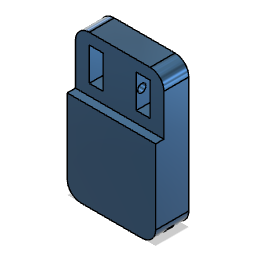
Robot Assembly Prototype v7 (Autodesk Fusion 360 archive; units mm, degrees)
design "Draft Sketch"
Autodesk Fusion 360 part; units mm, degrees
sketch "Sketch1" plane through (0, 0, 0) normal (0, 0, 1) x (1, 0, 0)
  line L0 (0, 0) -> (-320, 0)
  line L1 (-320, 0) -> (-320, 320)
  line L2 (-320, 320) -> (0, 320)
  line L3 (0, 320) -> (0, 0)
  line L4 (-320, 320) -> (-320, 470)
  line L5 (-270, 520) -> (-50, 520)
  line L6 (0, 470) -> (0, 320)
  arc A0 (-270, 520) -> (-320, 470) centre (-270, 470) ccw
  arc A1 (0, 470) -> (-50, 520) centre (-50, 470) ccw
  point P0 (-320, 520)
  dimension "d1" = 320
  dimension "d2" = 320
  dimension "d3" = 200
  dimension "d4" = 50
  dimension "d5" = 50
  constraint coincident L0.start L3.end
  constraint horizontal L0
  constraint perpendicular L0 L1
  constraint perpendicular L1 L2
  constraint perpendicular L0 L3
  constraint perpendicular L2 L4
  constraint perpendicular L4 L5
  constraint perpendicular L2 L6
  constraint coincident P0 L4
  constraint coincident P0 L5
  constraint tangent L4 A0
  constraint tangent L5 A0
  constraint tangent L5 A1
  constraint tangent L6 A1
  measures "d1" distance of L0.start L0.end
  measures "d2" distance of L0.end L1.end
  measures "d3" distance of L1.end P0
  measures "d4" radius of A0
  measures "d5" radius of A1
extrude "Extrude1" add sketch "Sketch1" along normal blind 70 contours L2 L4 L5 L6 A0 A1
extrude "Extrude2" add sketch "Sketch1" along normal blind 100 contours L0 L1 L2 L3
sketch "Sketch2" plane through (0, 0, 0) normal (1, 0, 0) x (0, 0, -1)
sketch "Sketch3" plane through (0, 0, 0) normal (1, 0, 0) x (0, 0, -1)
  line L0 (-70, 320) -> (-70, 390)
  circle A0 centre (-50, 390) radius 50
  dimension "d10" = 70
  dimension "d11" = 100
  constraint vertical L0
  measures "d10" distance of L0.start L0.end
  measures "d11" diameter of A0
extrude "Extrude3" add sketch "Sketch3" against normal blind 30
sketch "Sketch4" plane through (-320, 0, 0) normal (-1, 0, 0) x (0, 0, 1)
  line L0 (0, 470) -> (0, 0)
  line L1 (0, 0) -> (100, 0)
  line L2 (100, 0) -> (100, 320)
  line L3 (100, 320) -> (70, 320)
  line L4 (70, 320) -> (70, 470)
  line L5 (70, 470) -> (0, 470)
  line L6 (70, 320) -> (70, 390)
  circle A0 centre (50, 390) radius 50
  dimension "d14" = 70
  constraint coincident L3.end L4.start
  constraint perpendicular L3 L6
  measures "d14" distance of L3.end L6.end
extrude "Extrude4" add sketch "Sketch4" against normal blind 30 contours L4 L6 A0 picked at (89.8253, 392.4067)
delete_face "DeleteFace1" 1 faces at (-290, 381.5611, 84.673)
delete_face "DeleteFace2" 1 faces at (-10, 346.317, 74.3269)
sketch "Sketch5" plane through (0, 0, 0) normal (0, 0, 1) x (1, 0, 0)
sketch "Sketch6" plane through (0, 0, 0) normal (0, 0, 1) x (1, 0, 0)
sketch "Sketch7" plane through (0, 0, 0) normal (0, 0, 1) x (1, 0, 0)
sketch "Sketch8" plane through (0, 0, 70) normal (0, 0, 1) x (1, 0, 0)
  line L0 (-320, 320) -> (0, 320)
  line L1 (0, 320) -> (0, 470)
  arc A0 (0, 470) -> (-50, 520) centre (-50, 470) ccw
  line L2 (-50, 520) -> (-270, 520)
  arc A1 (-270, 520) -> (-320, 470) centre (-270, 470) ccw
  line L3 (-320, 470) -> (-320, 320)
  line L4 (-220, 420) -> (-220, 460)
  line L5 (-220, 460) -> (-280, 460)
  line L6 (-280, 460) -> (-280, 380)
  line L7 (-280, 380) -> (-220, 380)
  line L8 (-220, 380) -> (-220, 420)
  line L9 (-100, 420) -> (-100, 460)
  line L10 (-100, 460) -> (-40, 460)
  line L11 (-40, 460) -> (-40, 380)
  line L12 (-40, 380) -> (-100, 380)
  line L13 (-100, 380) -> (-100, 420)
  dimension "d19" = 40
  dimension "d20" = 60
  constraint perpendicular L4 L5
  constraint perpendicular L6 L7
  constraint perpendicular L9 L10
  constraint perpendicular L10 L11
  constraint perpendicular L9 L12
  measures "d19" distance of L4.start L4.end
  measures "d20" distance of L4.end L5.end
extrude "Extrude5" cut sketch "Sketch8" against normal blind 40 contours L4 L5 L6 L7 L8
extrude "Extrude6" cut sketch "Sketch8" against normal blind 40 contours L9 L10 L11 L12 L13
hole "Hole1" at (-100, 420, 50) direction (-1, 0, 0) diameter 30 depth 140 tip angle 118
extrude "Extrude7" cut 1 faces at (-80, 433.3333, 30) along direction (0, 0, -1) blind 10
extrude "Extrude8" cut 1 faces at (-240, 406.6667, 30) along direction (0, 0, -1) blind 10
sketch "Sketch9" plane through (0, 520, 0) normal (0, 1, 0) x (-1, 0, 0)
  line L0 (50, 0) -> (270, 0)
  line L1 (270, 0) -> (270, 70)
  line L2 (270, 70) -> (50, 70)
  line L3 (50, 70) -> (50, 0)
  line L4 (172, 35) -> (172, 23)
  line L5 (172, 35) -> (172, 47)
  line L6 (172, 47) -> (148, 47)
  line L7 (148, 47) -> (148, 23)
  line L8 (148, 23) -> (172, 23)
sketch "Sketch10" plane through (0, 0, 0) normal (0, 0, 1) x (1, 0, 0)
sketch "Sketch11" plane through (0, 520, 0) normal (0, 1, 0) x (-1, 0, 0)
  line L0 (50, 0) -> (270, 0)
  line L1 (270, 0) -> (270, 70)
  line L2 (270, 70) -> (50, 70)
  line L3 (50, 70) -> (50, 0)
sketch "Sketch12" plane through (0, 520, 0) normal (0, 1, 0) x (-1, 0, 0)
fillet "Fillet1" radius 50 1 edges at (0, 0, 50)
fillet "Fillet2" radius 50 1 edges at (-320, 0, 50)
extrude "Extrude10" add sketch "Sketch1" against normal blind 20 contours L2 L4 L5 L6 A0 A1
extrude "Extrude11" add 1 faces at (-223.3333, 203.5956, 0) along direction (0, 0, -1) blind 20
extrude "Extrude12" cut 1 faces at (-240, 406.6667, 20) along direction (0, 0, -1) blind 30
extrude "Extrude13" cut 1 faces at (-80, 433.3333, 20) along direction (0, 0, -1) blind 30
extrude "Extrude14" cut 1 faces at (-240, 460, 43.3333) along direction (0, 1, 0) blind 20
extrude "Extrude15" cut 1 faces at (-260, 380, 43.3333) along direction (0, -1, 0) blind 20
extrude "Extrude16" cut 1 faces at (-80, 460, 43.3333) along direction (0, 1, 0) blind 20
extrude "Extrude17" cut 1 faces at (-60, 380, 43.3333) along direction (0, -1, 0) blind 20
sketch "Sketch13" plane through (0, 0, 0) normal (0, 1, 0) x (1, 0, 0)
  line L0 (-160, -52) -> (-148, -52)
  line L1 (-148, -52) -> (-148, -28)
  line L2 (-148, -28) -> (-172, -28)
  line L3 (-172, -28) -> (-172, -52)
  line L4 (-172, -52) -> (-160, -52)
  dimension "d91" = 12
  dimension "d92" = 24
  dimension "d93" = 24
  dimension "d94" = 24
  dimension "d95" = 12
  constraint perpendicular L0 L1
  constraint perpendicular L1 L2
  constraint perpendicular L0 L3
  constraint perpendicular L1 L4
  measures "d91" distance of L0.start L0.end
  measures "d92" distance of L0.end L1.end
  measures "d93" distance of L1.end L2.end
  measures "d94" distance of L2.end L3.end
  measures "d95" distance of L3.end L0.start
extrude "Extrude18" cut sketch "Sketch13" along normal blind 10
ref_plane "WorkPlane1" through (-9.8857, 20.153, 31.144) normal (0.802286, -0.59694, 0) x (-0.59694, -0.802286, 0)
sketch "Sketch14" plane through (-9.8857, 20.153, 31.144) normal (0.802286, -0.59694, 0) x (-0.59694, -0.802286, 0)
  line L0 (5, -20) -> (-7, -20)
  line L1 (-7, -20) -> (-7, 4)
  line L2 (-7, 4) -> (17, 4)
  line L3 (17, 4) -> (17, -20)
  line L4 (17, -20) -> (5, -20)
  dimension "d102" = 12
  dimension "d103" = 24
  dimension "d104" = 24
  dimension "d105" = 24
  dimension "d106" = 12
  constraint perpendicular L1 L2
  measures "d102" distance of L0.start L0.end
  measures "d103" distance of L0.end L1.end
  measures "d104" distance of L1.end L2.end
  measures "d105" distance of L2.end L3.end
  measures "d106" distance of L3.end L0.start
extrude "Extrude19" cut sketch "Sketch14" against normal blind 10
ref_plane "WorkPlane2" through (-307.0527, 16.4278, 56.3835) normal (-0.741055, -0.671444, 0) x (-0.671444, 0.741055, 0)
sketch "Sketch15" plane through (-307.0527, 16.4278, 56.3835) normal (-0.741055, -0.671444, 0) x (-0.671444, 0.741055, 0)
  line L0 (10.5209, 16.4074) -> (10.5209, 4.4074)
  line L1 (10.5209, 4.4074) -> (-13.4791, 4.4074)
  line L2 (-13.4791, 4.4074) -> (-13.4791, 28.4074)
  line L3 (-13.4791, 28.4074) -> (10.5209, 28.4074)
  line L4 (10.5209, 28.4074) -> (10.5209, 16.4074)
  dimension "d113" = 12
  dimension "d114" = 24
  dimension "d115" = 24
  dimension "d116" = 24
  dimension "d117" = 12
  measures "d113" distance of L0.start L0.end
  measures "d114" distance of L0.end L1.end
  measures "d115" distance of L1.end L2.end
  measures "d116" distance of L2.end L3.end
  measures "d117" distance of L3.end L0.start
extrude "Extrude20" cut sketch "Sketch15" against normal blind 10
extrude "Extrude21" add 1 faces at (-280, 440, 43.3333) along direction (1, 0, 0) blind 10
extrude "Extrude22" add 1 faces at (-40, 440, 43.3333) along direction (-1, 0, 0) blind 10
move_body "Move1" bodies 1 to x (1, 0, 0) y (0, 1, 0) z (0, 0, 1) at (160, 0, -100)
move_body "Move2" bodies 1 to x (1, 0, 0) y (0, 1, 0) z (0, 0, 1) at (0, 0, 60)

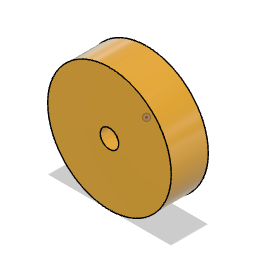
design "Wheel"
Autodesk Fusion 360 part; units mm, degrees
sketch "Sketch1" plane through (0, 0, 0) normal (0, 0, 1) x (1, 0, 0)
  circle A0 centre (0, 0) radius 7.5
  dimension "d2" = 15
  measures "d2" diameter of A0
sketch "Sketch2" plane through (0, 0, 0) normal (0, 0, 1) x (1, 0, 0)
sketch "Sketch3" plane through (0, 0, 0) normal (0, 0, 1) x (1, 0, 0)
  circle A0 centre (0, 0) radius 30
  dimension "d4" = 60
  constraint coincident A0.centre origin
  measures "d4" diameter of A0
extrude "Extrude1" add sketch "Sketch3" along normal blind 5
extrude "Extrude2" cut sketch "Sketch1" along normal blind 5
sketch "Sketch4" plane through (0, 0, 5) normal (0, 0, 1) x (1, 0, 0)
  circle A0 centre (0, 0) radius 7.5
  circle A1 centre (0, 0) radius 30
extrude "Extrude3" add sketch "Sketch4" along normal blind 5
extrude "Extrude4" add 1 faces at (22.3604, -1.863, 10) along direction (0, 0, 1) blind 5
sketch "Sketch5" plane through (0, 0, 15) normal (0, 0, 1) x (1, 0, 0)
  circle A0 centre (0, 0) radius 7.5
  circle A1 centre (0, 0) radius 30
  circle A2 centre (0, 0) radius 50
  dimension "d13" = 100
  constraint coincident A0.centre A1.centre
  measures "d13" diameter of A2
extrude "Extrude5" add sketch "Sketch5" against normal blind 15 contours A2
extrude "Extrude6" add 1 faces at (35.6193, -2.8566, 15) along direction (0, 0, 1) blind 15

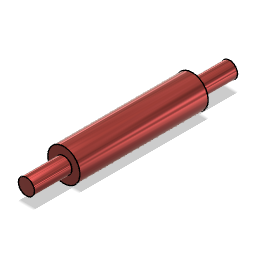
design "rod"
Autodesk Fusion 360 part; units mm, degrees
sketch "Sketch1" plane through (0, 0, 0) normal (0, 0, 1) x (1, 0, 0)
  circle A0 centre (0, 0) radius 15
  dimension "d1" = 30
  constraint coincident A0.centre origin
  measures "d1" diameter of A0
extrude "Extrude1" add sketch "Sketch1" along normal blind 120
sketch "Sketch2" plane through (0, 0, 120) normal (0, 0, 1) x (1, 0, 0)
  circle A0 centre (0, 0) radius 15
  circle A1 centre (0, 0) radius 7.5
  dimension "d4" = 15
  constraint concentric A0 A1
  measures "d4" diameter of A1
extrude "Extrude2" add sketch "Sketch2" along normal blind 10 contours A1
sketch "Sketch3" plane through (0, 0, 0) normal (0, 0, 1) x (1, 0, 0)
  circle A0 centre (0, 0) radius 7.5
  dimension "d7" = 15
  constraint coincident A0.centre origin
  measures "d7" diameter of A0
extrude "Extrude3" add sketch "Sketch3" against normal blind 10
extrude "Extrude4" add 1 faces at (1.9158, 2.8099, 130) along direction (0, 0, 1) blind 10
extrude "Extrude5" add 1 faces at (1.9158, 2.8099, -10) along direction (0, 0, -1) blind 10
extrude "Extrude6" add 1 faces at (1.9158, 2.8099, 140) along direction (0, 0, 1) blind 15
extrude "Extrude7" add 1 faces at (1.9158, 2.8099, -20) along direction (0, 0, -1) blind 15
